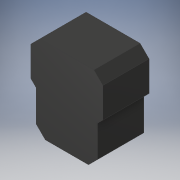
# Autodesk Inventor part: XT-LG-05
Saved by Autodesk Inventor 2017 SP1 (Build 210196100, 196)
## iProperties
Created: 2019-11-11
Part Number: XT-LG-05
Material: ABS Plastic
Document SubType Name: Modeling
Designer: Zach
Density: 1.06 g/cm^3
Appearance: Smooth - Black
Author: Zach
Autodesk Inventor part; units mm, degrees
ref_plane "YZ Plane" through (0, 0, 0) normal (1, 0, 0) x (0, 1, 0)
ref_plane "XZ Plane" through (0, 0, 0) normal (0, 1, 0) x (-1, 0, 0)
ref_plane "XY Plane" through (0, 0, 0) normal (0, 0, 1) x (1, 0, 0)
sketch "Sketch1" plane through (0, 0, 0) normal (0, 0, 1) x (1, 0, 0)
  line L0 (-60.1273, 59) -> (60.1273, 59)
  line L1 (-60.1273, 59) -> (-80.1273, 39)
  line L2 (-80.1273, 39) -> (-80.1273, -28)
  line L3 (-68.1273, -40) -> (-80.1273, -28)
  line L4 (-68.1273, -110) -> (-68.1273, -40)
  line L5 (-68.1273, -110) -> (-48.1273, -130)
  line L6 (-48.1273, -130) -> (48.1273, -130)
  line L7 (48.1273, -130) -> (68.1273, -110)
  line L8 (68.1273, -40) -> (68.1273, -110)
  line L9 (80.1273, -28) -> (68.1273, -40)
  line L10 (80.1273, 39) -> (80.1273, -28)
  line L11 (60.1273, 59) -> (80.1273, 39)
  point P0 (0, 0)
  point P1 (0, 0)
  constraints: 24 end point
extrude "Extrusion1" add sketch "Sketch1" along normal blind 3
sketch "Sketch2" plane through (0, 0, 0) normal (0, 0, -1) x (-1, 0, 0)
  line L0 (60.1273, 59) -> (-60.1273, 59) projected
  line L1 (-60.1273, 59) -> (-80.1273, 39) projected
  line L2 (-80.1273, 39) -> (-80.1273, -28) projected
  line L3 (-80.1273, -28) -> (-68.1273, -40) projected
  line L4 (-68.1273, -40) -> (-68.1273, -110) projected
  line L5 (-68.1273, -110) -> (-48.1273, -130) projected
  line L6 (-48.1273, -130) -> (48.1273, -130) projected
  line L7 (48.1273, -130) -> (68.1273, -110) projected
  line L8 (68.1273, -110) -> (68.1273, -40) projected
  line L9 (68.1273, -40) -> (80.1273, -28) projected
  line L10 (80.1273, -28) -> (80.1273, 39) projected
  line L11 (80.1273, 39) -> (60.1273, 59) projected
  line L12 (-59.2575, 56.9) -> (59.2575, 56.9)
  line L13 (59.2575, 56.9) -> (78.0273, 38.1302)
  line L14 (78.0273, 38.1302) -> (78.0273, -27.1302)
  line L15 (78.0273, -27.1302) -> (66.0273, -39.1302)
  line L16 (66.0273, -39.1302) -> (66.0273, -109.1302)
  line L17 (66.0273, -109.1302) -> (47.2575, -127.9)
  line L18 (47.2575, -127.9) -> (-47.2575, -127.9)
  line L19 (-47.2575, -127.9) -> (-66.0273, -109.1302)
  line L20 (-66.0273, -109.1302) -> (-66.0273, -39.1302)
  line L21 (-66.0273, -39.1302) -> (-78.0273, -27.1302)
  line L22 (-78.0273, -27.1302) -> (-78.0273, 38.1302)
  line L23 (-78.0273, 38.1302) -> (-59.2575, 56.9)
  point P0 (0, 0)
  dimension "d2" = 2.1
  constraints: 24 end point, 11 other
  measures "d2" distance between parallel lines of L0 L12
extrude "Extrusion2" add sketch "Sketch2" along normal blind 100
body "Solid1"
